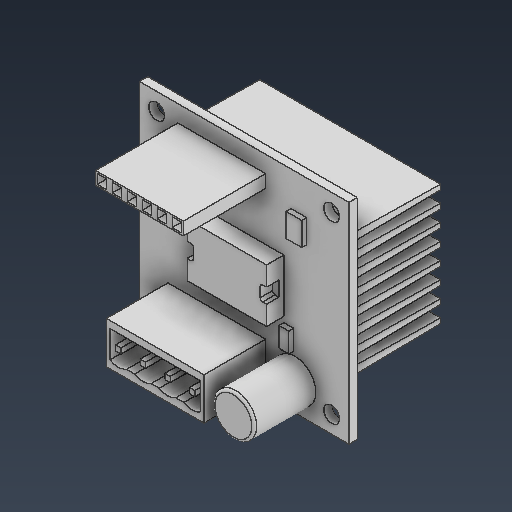
# Autodesk Inventor part: IBTMini
Saved by Autodesk Inventor 2025.2 (Build 292293000, 293)
## iProperties
Created: 2023-12-09
Part Number: IBTMini
Material: Generic
Document SubType Name: Modeling
Designer: valer
Density: 1 g/cm^3
Appearance: Default
Author: valer
Autodesk Inventor part; units mm, degrees
ref_plane "YZ Plane" through (0, 0, 0) normal (1, 0, 0) x (0, 1, 0)
ref_plane "XZ Plane" through (0, 0, 0) normal (0, 1, 0) x (-1, 0, 0)
ref_plane "XY Plane" through (0, 0, 0) normal (0, 0, 1) x (1, 0, 0)
sketch "Sketch1" plane through (0, 0, 0) normal (0, 0, 1) x (1, 0, 0)
  line L0 (-21.25, 21.25) -> (21.25, 21.25)
  line L1 (21.25, 21.25) -> (21.25, -21.25)
  line L2 (21.25, -21.25) -> (-21.25, -21.25)
  line L3 (-21.25, -21.25) -> (-21.25, 21.25)
  line L4 (-29.75, 0) -> (29.75, 0) construction
  line L5 (0, -29.75) -> (0, 29.75) construction
  point P0 (0, 0)
  point P1 (0, 21.25)
  point P2 (-21.25, 0)
  dimension "d0" = 42.5
  constraints: 8 end point, 2 midpoint, 2 parallel, 2 perpendicular, 2 point on line, 1 horizontal
  measures "d0" distance of L0.start L0.end
extrude "Extrusion1" add sketch "Sketch1" along normal blind 1.7
sketch "Sketch2" plane through (0, 0, 1.7) normal (0, 0, 1) x (1, 0, 0)
  circle A0 centre (-17.75, 17.75) radius 3.5 construction
  line L0 (21.25, 21.25) -> (-21.25, 21.25) construction
  line L1 (-21.25, 21.25) -> (-21.25, -21.25) construction
  circle A1 centre (-17.75, 17.75) radius 1.6
  line L2 (-17.75, 19.35) -> (-17.75, 21.25) construction
  line L3 (-19.35, 17.75) -> (-21.25, 17.75) construction
  line L4 (-29.75, 0) -> (29.75, 0) construction
  line L5 (0, -29.75) -> (0, 29.75) construction
  circle A2 centre (17.75, 17.75) radius 1.6
  circle A3 centre (-17.75, -17.75) radius 1.6
  circle A4 centre (17.75, -17.75) radius 1.6
  point P0 (0, 0)
  dimension "d3" = 1.9
  dimension "d4" = 3.2
  constraints: 5 centre point, 4 end point, 4 point on circle, 3 perpendicular, 3 symmetric about line, 2 point on line, 2 tangent, 1 coincident, 3 other
  measures "d3" distance of L2.start L2.end
  measures "d4" diameter of A1
extrude "Extrusion2" cut sketch "Sketch2" against normal blind 1.7
sketch "Sketch3" plane through (0, 0, 1.7) normal (0, 0, 1) x (1, 0, 0)
  line L0 (-21.25, 21.25) -> (-21.25, -21.25) construction
  line L1 (-21.25, 0) -> (21.25, 0) construction
  line L2 (21.25, -21.25) -> (21.25, 21.25) construction
  line L3 (-8.05, 5.4) -> (8.05, 5.4)
  line L4 (8.05, 5.4) -> (8.05, -5.4)
  line L5 (8.05, -5.4) -> (-8.05, -5.4)
  line L6 (-8.05, -5.4) -> (-8.05, 5.4)
  line L7 (0, -29.75) -> (0, 29.75) construction
  point P0 (0, 0)
  point P1 (-8.05, 0)
  point P2 (0, 5.4)
  dimension "d7" = 16.1
  dimension "d8" = 10.8
  constraints: 10 end point, 4 midpoint, 2 parallel, 2 point on line, 1 horizontal, 1 perpendicular
  measures "d7" distance of L3.start L3.end
  measures "d8" distance of L3.end L4.end
extrude "Extrusion3" add sketch "Sketch3" along normal blind 3.5
sketch "Sketch4" plane through (0, 0, 5.2) normal (0, 0, 1) x (1, 0, 0)
  line L0 (-8.05, -5.4) -> (8.05, -5.4) projected
  line L1 (8.05, -5.4) -> (8.05, 5.4) projected
  line L2 (8.05, 5.4) -> (-8.05, 5.4) projected
  line L3 (-8.05, 5.4) -> (-8.05, -5.4) projected
  line L4 (6.75, 1.5) -> (8.05, 1.5)
  line L5 (8.05, 1.5) -> (8.05, -1.5)
  line L6 (8.05, -1.5) -> (6.75, -1.5)
  line L7 (6.75, -1.5) -> (6.75, 1.5)
  line L8 (0, -29.75) -> (0, 29.75) construction
  line L9 (-6.75, 1.5) -> (-8.05, 1.5)
  line L10 (-8.05, 1.5) -> (-8.05, -1.5)
  line L11 (-8.05, -1.5) -> (-6.75, -1.5)
  line L12 (-6.75, -1.5) -> (-6.75, 1.5)
  point P0 (0, 0)
  point P1 (8.05, 0)
  dimension "d11" = 3
  dimension "d12" = 1.3
  constraints: 16 end point, 4 symmetric about line, 2 midpoint, 2 parallel, 1 horizontal, 1 perpendicular
  measures "d11" distance of L6.end L4.start
  measures "d12" distance of L5.end L6.end
extrude "Extrusion4" cut sketch "Sketch4" against normal blind 2.5 contours L3 L9 L12 L11 | L6 L7 L4 L1
fillet "Fillet1" radius 0.5 4 edges at (6.75, 1.5, 3.95) (6.75, -1.5, 3.95) (-6.75, 1.5, 3.95) (-6.75, -1.5, 3.95)
sketch "Sketch5" plane through (0, 0, 1.7) normal (0, 0, 1) x (1, 0, 0)
  circle A0 centre (10.3, -15.5) radius 4.25
  line L0 (-15.45, -11.25) -> (4.35, -11.25)
  line L1 (4.35, -11.25) -> (4.35, -19.75)
  line L2 (4.35, -19.75) -> (-15.45, -19.75)
  line L3 (-15.45, -19.75) -> (-15.45, -11.25)
  line L4 (-13.45, 17.85) -> (4.35, 17.85)
  line L5 (4.35, 17.85) -> (4.35, 15.25)
  line L6 (4.35, 15.25) -> (-13.45, 15.25)
  line L7 (-13.45, 15.25) -> (-13.45, 17.85)
  line L8 (21.25, 21.25) -> (-21.25, 21.25) projected
  line L9 (-21.25, 21.25) -> (-21.25, -21.25) projected
  line L10 (-15.45, -15.5) -> (14.55, -15.5) construction
  line L11 (4.35, -11.25) -> (10.3, -11.25) construction
  line L12 (-21.25, -21.25) -> (21.25, -21.25) construction
  line L13 (21.25, -21.25) -> (21.25, 21.25) projected
  point P0 (0, 0)
  point P1 (-13.45, 16.55)
  dimension "d16" = 17.8
  dimension "d17" = 2.6
  dimension "d18" = 7.8
  dimension "d19" = 3.4
  dimension "d20" = 30
  dimension "d21" = 8.5
  dimension "d22" = 1.5
  dimension "d23" = 6.7
  constraints: 20 end point, 5 parallel, 2 horizontal, 2 midpoint, 2 perpendicular, 2 point on circle, 2 point on line, 1 centre point, 1 collinear, 1 tangent
  measures "d16" distance of L5.end L6.end
  measures "d17" distance of L4.end L5.end
  measures "d18" distance from line of L9 point (-13.45, 16.55)
  measures "d19" distance between parallel lines of L8 L4
  measures "d20" distance of L10.end L10.start
  measures "d21" distance of L2.end L0.start
  measures "d22" distance between parallel lines of L12 L2
  measures "d23" distance from line of L13 L10.end
extrude "Extrusion5" add sketch "Sketch5" along normal blind 12.5 contours A0 | L0 L1 L2 L3
extrude "Extrusion6" add sketch "Sketch5" along normal blind 16.7 contours L4 L5 L6 L7
sketch "Sketch6" plane through (0, 0, 14.2) normal (0, 0, 1) x (1, 0, 0)
  line L0 (-15.45, -19.75) -> (-15.45, -11.25) construction
  line L1 (-15.45, -15.5) -> (4.35, -15.5) construction
  line L2 (4.35, -11.25) -> (4.35, -19.75) construction
  line L3 (-13.5913, -14.9587) -> (-12.5087, -14.9587)
  line L4 (-12.5087, -14.9587) -> (-12.5087, -16.0413)
  line L5 (-12.5087, -16.0413) -> (-13.5913, -16.0413)
  line L6 (-13.5913, -16.0413) -> (-13.5913, -14.9587)
  line L7 (-7.5087, -14.9587) -> (-7.5087, -16.0413)
  line L8 (-8.5913, -14.9587) -> (-7.5087, -14.9587)
  line L9 (-8.5913, -16.0413) -> (-8.5913, -14.9587)
  line L10 (-7.5087, -16.0413) -> (-8.5913, -16.0413)
  line L11 (-2.5087, -14.9587) -> (-2.5087, -16.0413)
  line L12 (-3.5913, -14.9587) -> (-2.5087, -14.9587)
  line L13 (-3.5913, -16.0413) -> (-3.5913, -14.9587)
  line L14 (-2.5087, -16.0413) -> (-3.5913, -16.0413)
  line L15 (2.4913, -14.9587) -> (2.4913, -16.0413)
  line L16 (1.4087, -14.9587) -> (2.4913, -14.9587)
  line L17 (1.4087, -16.0413) -> (1.4087, -14.9587)
  line L18 (2.4913, -16.0413) -> (1.4087, -16.0413)
  line L19 (-14.73, -12.65) -> (3.63, -12.65)
  line L20 (3.63, -12.65) -> (3.63, -18.15)
  line L21 (3.63, -18.15) -> (-14.73, -18.15)
  line L22 (-14.73, -18.15) -> (-14.73, -12.65)
  line L23 (4.35, -11.25) -> (-15.45, -11.25) construction
  line L24 (-15.45, -19.75) -> (4.35, -19.75) construction
  line L25 (-5.55, -12.65) -> (-5.55, -18.15) construction
  line L26 (-10.55, -18.15) -> (-10.55, -12.65) construction
  line L27 (-0.55, -18.15) -> (-0.55, -12.65) construction
  line L28 (-13.5913, -14.9587) -> (-12.5087, -16.0413) construction
  circle A0 centre (-13.05, -15.5) radius 3.1377 construction
  line L29 (-11.37, -18.15) -> (-11.37, -19.75) construction
  line L30 (4.35, -19.75) -> (-15.45, -19.75) projected
  arc A1 (-14.73, -18.15) -> (-11.37, -18.15) centre (-13.05, -15.5) ccw
  arc A2 (-9.73, -18.15) -> (-6.37, -18.15) centre (-8.05, -15.5) ccw
  arc A3 (-4.73, -18.15) -> (-1.37, -18.15) centre (-3.05, -15.5) ccw
  arc A4 (0.27, -18.15) -> (3.63, -18.15) centre (1.95, -15.5) ccw
  point P0 (0, 0)
  point P1 (-13.5913, -15.5)
  point P2 (-8.5913, -15.5)
  point P3 (-3.5913, -15.5)
  point P4 (1.4087, -15.5)
  point P5 (-9.73, -18.15)
  point P6 (-1.37, -18.15)
  point P7 (0.27, -18.15)
  dimension "d30" = 5
  dimension "d35" = 1.8587
  dimension "d36" = 1.8587
  dimension "d37" = 1.4
  dimension "d38" = 0.72
  dimension "d39" = 1.6
  dimension "d40" = 0.72
  dimension "d41" = 4.18
  dimension "d43" = 1.9587
  dimension "d44" = 1.9587
  constraints: 52 end point, 10 point on circle, 10 symmetric about line, 6 midpoint, 5 centre point, 5 perpendicular, 5 point on line, 4 parallel, 3 horizontal, 1 concentric, 30 other
  measures "d30" distance of L3.end L7.start
  measures "d35" distance between parallel lines of L0 L6
  measures "d36" distance between parallel lines of L2 L15
  measures "d37" distance between parallel lines of L23 L19
  measures "d38" distance between parallel lines of L0 L22
  measures "d39" distance between parallel lines of L24 L21
  measures "d40" distance between parallel lines of L2 L20
  measures "d41" distance between parallel lines of L22 L26
  measures "d43" distance between parallel lines of L9 L26
  measures "d44" distance from line of L4.end L26
extrude "Extrusion7" cut sketch "Sketch6" against normal up to surface (12.5 mm away)
fillet "Fillet2" radius 0.5 1 edges at (6.05, -15.5, 14.2)
sketch "Sketch7" plane through (0, 0, 18.4) normal (0, 0, 1) x (1, 0, 0)
  line L0 (-13.45, 15.25) -> (4.35, 15.25) projected
  line L1 (4.35, 15.25) -> (4.35, 17.85) projected
  line L2 (4.35, 17.85) -> (-13.45, 17.85) projected
  line L3 (-13.45, 17.85) -> (-13.45, 15.25) projected
  line L4 (-13.1, 17.5) -> (4, 17.5)
  line L5 (4, 17.5) -> (4, 15.6)
  line L6 (4, 15.6) -> (-13.1, 15.6)
  line L7 (-13.1, 15.6) -> (-13.1, 17.5)
  line L8 (-11.2, 17.5) -> (-11.2, 15.6)
  line L9 (4.35, 15.25) -> (-13.45, 15.25) projected
  line L10 (-4.55, 15.25) -> (-4.55, 17.85) construction
  line L11 (-13.45, 17.85) -> (4.35, 17.85) projected
  line L12 (2.1, 17.5) -> (2.1, 15.6)
  line L13 (-11.2, 16.55) -> (2.1, 16.55) construction
  line L14 (-10.06, 17.5) -> (-8.16, 17.5)
  line L15 (-8.16, 17.5) -> (-8.16, 15.6)
  line L16 (-8.16, 15.6) -> (-10.06, 15.6)
  line L17 (-10.06, 15.6) -> (-10.06, 17.5)
  line L18 (-7.02, 17.5) -> (-5.12, 17.5)
  line L19 (-5.12, 17.5) -> (-5.12, 15.6)
  line L20 (-5.12, 15.6) -> (-7.02, 15.6)
  line L21 (-7.02, 15.6) -> (-7.02, 17.5)
  line L22 (-3.98, 17.5) -> (-2.08, 17.5)
  line L23 (-2.08, 17.5) -> (-2.08, 15.6)
  line L24 (-2.08, 15.6) -> (-3.98, 15.6)
  line L25 (-3.98, 15.6) -> (-3.98, 17.5)
  line L26 (-0.94, 17.5) -> (0.96, 17.5)
  line L27 (0.96, 17.5) -> (0.96, 15.6)
  line L28 (0.96, 15.6) -> (-0.94, 15.6)
  line L29 (-0.94, 15.6) -> (-0.94, 17.5)
  point P0 (0, 0)
  point P1 (0.96, 17.5)
  dimension "d49" = 0.35
  dimension "d50" = 1.9
  dimension "d51" = 1.9
  dimension "d52" = 1.9
  dimension "d53" = 1.14
  dimension "d54" = 1.14
  dimension "d55" = 1.14
  dimension "d56" = 1.14
  dimension "d57" = 1.14
  constraints: 48 end point, 11 collinear, 8 parallel, 5 perpendicular, 4 horizontal, 4 midpoint, 2 point on line, 2 symmetric about line, 3 other
  measures "d49" distance between parallel lines of L2 L4
  measures "d50" distance of L6.end L4.start
  measures "d51" distance between parallel lines of L7 L8
  measures "d52" distance between parallel lines of L15 L17
  measures "d53" distance between parallel lines of L17 L8
  measures "d54" distance between parallel lines of L21 L15
  measures "d55" distance between parallel lines of L25 L19
  measures "d56" distance between parallel lines of L29 L23
  measures "d57" distance between parallel lines of L12 L27
extrude "Extrusion8" cut sketch "Sketch7" against normal up to surface (16.7 mm away) contours L4 L8 L6 L7 | L4 L15 L6 L17 | L4 L19 L6 L21 | L4 L23 L6 L25 | L4 L27 L6 L29 | L4 L5 L6 L12
sketch "Sketch8" plane through (0, 0, 1.7) normal (0, 0, 1) x (1, 0, 0)
  line L0 (9.525, 9.525) -> (12.7, 9.525)
  line L1 (12.7, 9.525) -> (12.7, 14.2875)
  line L2 (12.7, 14.2875) -> (9.525, 14.2875)
  line L3 (9.525, 14.2875) -> (9.525, 9.525)
  point P0 (0, 0)
  dimension "d60" = 3.175
  dimension "d61" = 4.7625
  dimension "d62" = 12.7
  dimension "d63" = 14.2875
  constraints: 8 end point, 2 parallel, 1 horizontal, 1 perpendicular
  measures "d60" distance between parallel lines of L1 L3
  measures "d61" distance between parallel lines of L0 L2
  measures "d62" distance from line of point (0, 0) L1
  measures "d63" distance from line of point (0, 0) L2
extrude "Extrusion9" add sketch "Sketch8" along normal blind 1
sketch "Sketch9" plane through (0, 0, 0) normal (0, 0, -1) x (-1, 0, 0)
  line L0 (18.35, -12.55) -> (-18.35, -12.55)
  line L1 (-18.35, -12.55) -> (-18.35, 12.55)
  line L2 (-18.35, 12.55) -> (18.35, 12.55)
  line L3 (18.35, 12.55) -> (18.35, -12.55)
  line L4 (29.75, 0) -> (-29.75, 0) projected
  line L5 (0, -29.75) -> (0, 29.75) projected
  point P0 (0, 0)
  point P1 (0, -12.55)
  point P2 (18.35, 0)
  dimension "d66" = 25.1
  dimension "d67" = 36.7
  constraints: 8 end point, 2 midpoint, 2 parallel, 2 point on line, 1 horizontal, 1 perpendicular
  measures "d66" distance of L0.end L1.end
  measures "d67" distance of L0.start L0.end
extrude "Extrusion10" add sketch "Sketch9" along normal blind 19.8
sketch "Sketch11" plane through (0, 0, 1.7) normal (0, 0, 1) x (1, 0, 0)
  line L0 (8.05, -6.48) -> (10.05, -6.48)
  line L1 (10.05, -6.48) -> (10.05, -10.48)
  line L2 (10.05, -10.48) -> (8.05, -10.48)
  line L3 (8.05, -10.48) -> (8.05, -6.48)
  line L4 (21.25, -21.25) -> (21.25, 21.25) projected
  line L5 (-21.25, -21.25) -> (21.25, -21.25) projected
  point P0 (0, 0)
  point P1 (10.05, -8.48)
  dimension "d79" = 2
  dimension "d80" = 4
  dimension "d81" = 11.2
  dimension "d82" = 10.77
  constraints: 8 end point, 2 parallel, 1 horizontal, 1 midpoint, 1 perpendicular
  measures "d79" distance of L0.start L0.end
  measures "d80" distance of L0.end L1.end
  measures "d81" distance from line of L4 point (10.05, -8.48)
  measures "d82" distance between parallel lines of L5 L2
extrude "LedFeature" add sketch "Sketch11" along normal blind 1
sketch "Sketch12" plane through (18.35, -12.55, 0) normal (1, 0, 0) x (0, 0, -1)
  line L0 (0, -8.7) -> (0, 33.8) projected
  line L1 (0, 0) -> (19.8, 0) projected
  line L2 (2, 0) -> (2, 25.1)
  line L3 (0, 25.1) -> (19.8, 25.1) projected
  line L4 (2, 0) -> (19.8, 0.3)
  line L5 (19.8, 25.1) -> (19.8, 0) projected
  line L6 (19.8, 0.3) -> (19.8, 1.3)
  line L7 (19.8, 1.3) -> (2, 1.6)
  line L8 (19.8, 0.8) -> (2, 0.8) construction
  line L9 (2, 12.55) -> (19.8, 12.55) construction
  line L10 (2, 25.1) -> (19.8, 24.8)
  line L11 (19.8, 24.8) -> (19.8, 23.8)
  line L12 (19.8, 23.8) -> (2, 23.5)
  line L13 (2, 3.3571) -> (19.8, 3.6571)
  line L14 (19.8, 3.6571) -> (19.8, 4.6571)
  line L15 (19.8, 4.6571) -> (2, 4.9571)
  line L16 (19.8, 4.1571) -> (2, 4.1571) construction
  line L17 (2, 6.7143) -> (19.8, 7.0143)
  line L18 (19.8, 7.0143) -> (19.8, 8.0143)
  line L19 (19.8, 8.0143) -> (2, 8.3143)
  line L20 (19.8, 7.5143) -> (2, 7.5143) construction
  line L21 (2, 10.0714) -> (19.8, 10.3714)
  line L22 (19.8, 10.3714) -> (19.8, 11.3714)
  line L23 (19.8, 11.3714) -> (2, 11.6714)
  line L24 (19.8, 10.8714) -> (2, 10.8714) construction
  line L25 (2, 21.7429) -> (19.8, 21.4429)
  line L26 (19.8, 20.4429) -> (2, 20.1429)
  line L27 (2, 18.3857) -> (19.8, 18.0857)
  line L28 (19.8, 17.0857) -> (2, 16.7857)
  line L29 (2, 15.0286) -> (19.8, 14.7286)
  line L30 (19.8, 13.7286) -> (2, 13.4286)
  point P0 (0, 12.55)
  point P1 (2, 23.5)
  point P2 (2, 20.1429)
  point P3 (2, 16.7857)
  point P4 (2, 13.4286)
  dimension "d85" = 2
  dimension "d86" = 1.6
  dimension "d87" = 1
  dimension "d88" = 1.7571
  dimension "d89" = 1.7571
  dimension "d90" = 1.7571
  dimension "d91" = 0.8786
  dimension "d92" = 90.966
  dimension "d93" = 90.966
  dimension "d94" = 90.966
  dimension "d95" = 90.966
  dimension "d96" = 90.966
  dimension "d97" = 90.966
  constraints: 52 end point, 15 symmetric about line, 6 equal length, 4 horizontal, 4 midpoint, 2 point on line, 1 vertical, 24 other
  measures "d86" distance of L7.end L4.start
  measures "d87" distance of L6.end L4.end
  measures "d88" distance of L13.start L7.end
  measures "d89" distance of L17.start L15.end
  measures "d90" distance of L21.start L19.end
  measures "d91" distance of L9.start L23.end
extrude "Extrusion13" cut sketch "Sketch12" against normal through all contours L4 L5 L1 | L3 L5 L10 | L2 L13 L5 L7 | L12 L5 L25 L2 | L2 L17 L5 L15 | L26 L5 L27 L2 | L2 L21 L5 L19 | L28 L5 L29 L2 | L2 L30 L5 L23
equation "\"d36\" = d35"
equation "\"d40\" = d38"
equation "\"d44\" = d43"
equation "\"d51\" = d50"
equation "\"d52\" = d51"
equation "\"d54\" = d53"
equation "\"d55\" = d53"
equation "\"d56\" = d53"
equation "\"d57\" = d53"
equation "\"d89\" = d88"
equation "\"d90\" = d88"
equation "\"d91\" = 0.5 * d88"
equation "\"d93\" = d92"
equation "\"d95\" = d92"
equation "\"d96\" = d92"
equation "\"d97\" = d92"
body "Solid1"
